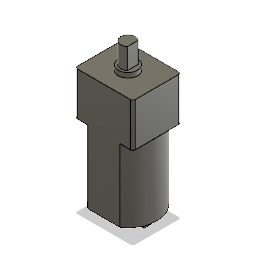
Motorized bigjoint (Autodesk Fusion 360 archive; units mm, degrees)
design "VE508 Small Gear Motor"
Autodesk Fusion 360 part; units mm, degrees
note: some values were not read from the file. Set by a fixed rule: which sketch regions a step uses.
(part 1 of 2)
sketch "Sketch1" plane through (0, 0, 0) normal (0, 1, 0) x (1, 0, 0) in component "Motor"
  line L0 (6, 5) -> (-6, 5)
  line L1 (-6, 5) -> (-6, -5)
  line L2 (-6, -5) -> (6, -5)
  line L3 (6, -5) -> (6, 5)
  line L4 (6, 5) -> (-6, -5) construction
  line L5 (-6, 5) -> (6, -5) construction
  dimension "d1" = 10
  dimension "d2" = 12
  constraint perpendicular L0 L1
  constraint parallel L0 L2
  constraint parallel L1 L3
  constraint horizontal L0
  constraint coincident L4 origin
  constraint coincident L5 origin
  measures "d1" distance of L0.end L1.end
  measures "d2" distance of L0.start L0.end
extrude "Extrude1" add sketch "Sketch1" against normal blind 9 makes body 1 in component "Motor"
sketch "Sketch2" plane through (0, -9, 0) normal (0, -1, 0) x (1, 0, 0) in component "Motor"
  line L0 (6, -5) -> (6, 5)
  line L1 (6, 5) -> (-6, 5)
  line L2 (-6, 5) -> (-6, -5)
  line L3 (-6, -5) -> (6, -5)
  circle A0 centre (0, 0) radius 6
  constraint coincident A0.centre origin
  constraint tangent L0 A0
extrude "Extrude2" add sketch "Sketch2" along normal blind 15 contours L1 L3 A0 bodies 1 in component "Motor"
sketch "Sketch3" plane through (0, -24, 0) normal (0, -1, 0) x (1, 0, 0) in component "Motor"
  arc A0 (3.3166, -5) -> (3.3166, 5) centre (0, 0) ccw
  line L0 (3.3166, 5) -> (-3.3166, 5)
  arc A1 (-3.3166, 5) -> (-3.3166, -5) centre (0, 0) ccw
  line L1 (-3.3166, -5) -> (3.3166, -5)
  circle A2 centre (0, 0) radius 2.5
  line L2 (-4, 0) -> (4, 0) construction
  line L3 (0, 5) -> (0, -5) construction
  line L4 (-4, 0.75) -> (-3.65, 0.75)
  line L5 (-3.65, 0.75) -> (-3.65, -0.75)
  line L6 (-3.65, -0.75) -> (-4, -0.75)
  line L7 (-4, -0.75) -> (-4, 0.75)
  line L8 (3.65, -0.75) -> (4, -0.75)
  line L9 (4, -0.75) -> (4, 0.75)
  line L10 (3.65, 0.75) -> (3.65, -0.75)
  line L11 (4, 0.75) -> (3.65, 0.75)
  dimension "d7" = 5
  dimension "d10" = 8
  dimension "d11" = 0.35
  dimension "d12" = 1.5
  constraint concentric A0 A2
  constraint horizontal L2
  constraint coincident A0.centre L2
  constraint midpoint L0 L3.start
  constraint midpoint L1 L3.end
  constraint symmetric L2.start L2.end L3
  constraint horizontal L4
  constraint vertical L5
  constraint horizontal L6
  constraint vertical L7
  constraint coincident L2.start L7
  constraint symmetric L2 L4 L6
  constraint symmetric L3 L4.start L9.end
  constraint symmetric L3 L4.end L10.start
  constraint symmetric L3 L5.end L8.start
  constraint symmetric L3 L6.end L8.end
  measures "d7" diameter of A2
  measures "d10" distance of L2.start L2.end
  measures "d11" distance of L5.end L6.end
  measures "d12" distance of L4.start L6.end
extrude "Extrude4" add sketch "Sketch3" along normal blind 2 contours L4 L5 L6 L7 | L8 L9 L10 L11 bodies 1 in component "Motor"
extrude "Extrude3" add sketch "Sketch3" along normal blind 1 contours A2 bodies 1 in component "Motor"
fillet "Fillet1" radius 0.5 4 edges at (6, -4.5, -5) (-6, -4.5, -5) (-6, -4.5, 5) (6, -4.5, 5) on bodies 1 in component "Motor"
sketch "Sketch4" plane through (0, 0, 0) normal (0, 1, 0) x (-1, 0, 0) in component "Motor"
  arc A0 (-5.5, 5) -> (-6, 4.5) centre (-5.5, 4.5) ccw
  line L0 (-6, 4.5) -> (-6, -4.5)
  arc A1 (-6, -4.5) -> (-5.5, -5) centre (-5.5, -4.5) ccw
  line L1 (-5.5, -5) -> (5.5, -5)
  arc A2 (5.5, -5) -> (6, -4.5) centre (5.5, -4.5) ccw
  line L2 (6, -4.5) -> (6, 4.5)
  arc A3 (6, 4.5) -> (5.5, 5) centre (5.5, 4.5) ccw
  line L3 (5.5, 5) -> (-5.5, 5)
  circle A4 centre (0, 0) radius 2
  dimension "d16" = 4
  constraint coincident A4.centre origin
  measures "d16" diameter of A4
extrude "Extrude5" add sketch "Sketch4" along normal blind 1 contours A4 bodies 1 in component "Motor"
sketch "Sketch5" plane through (0, 1, 0) normal (0, 1, 0) x (-1, 0, 0) in component "Motor"
  circle A0 centre (0, 0) radius 2
  circle A1 centre (0, 0) radius 1.5
  line L0 (-1, -1.118) -> (-1, 1.118)
  line L1 (3.3166, -5) -> (-3.3166, -5) construction
  line L2 (5.5, 5) -> (-5.5, 5) construction
  line L3 (1.5, -5) -> (1.5, 5) construction
  dimension "d19" = 3
  dimension "d20" = 2.5
  constraint concentric A0 A1
  constraint coincident A1 L0.start
  constraint coincident A1 L0.end
  constraint coincident L1 L3.start
  constraint coincident L2 L3.end
  constraint tangent A1 L3
  constraint perpendicular L2 L3
  measures "d19" diameter of A1
  measures "d20" distance of L0 L3
extrude "Extrude6" add sketch "Sketch5" along normal blind 4.3 separate body contours A1 L0 picked at (-0.4625, 0.4564) makes body 2 in component "Motor"
copy_body "CutPasteBodies1" bodies 2 removing the originals makes body 3 in component "Rotor"
component "Motor" placed x (1, 0, 0) y (0, 1, 0) z (0, 0, 1) at (0, 0, 0)
component "Rotor" placed x (1, 0, 0) y (0, 1, 0) z (0, 0, 1) at (0, 0, 0)

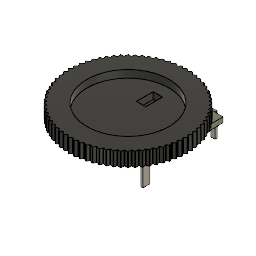
design "B503 Dial Potentiometer"
Autodesk Fusion 360 part; units mm, degrees
sketch "Sketch1" plane through (0, 0, 0) normal (0, 0, 1) x (1, 0, 0) in component "Knob"
  circle A0 centre (0, 0) radius 8
  circle A1 centre (0, 0) radius 7.75
  line L0 (0, 0) -> (8, 0) construction
  line L1 (7.7444, 0.2955) -> (7.9999, 0.04)
  line L2 (7.7444, -0.2955) -> (7.9999, -0.04)
  line L3 (7.7407, 0.3806) -> (7.9729, 0.6574)
  line L4 (7.6891, 0.9694) -> (7.966, 0.7371)
  line L5 (7.678, 1.0537) -> (7.8853, 1.3498)
  line L6 (7.5754, 1.6358) -> (7.8714, 1.4286)
  line L7 (7.557, 1.7189) -> (7.7377, 2.0319)
  line L8 (7.404, 2.2899) -> (7.717, 2.1092)
  line L9 (7.3784, 2.371) -> (7.5311, 2.6985)
  line L10 (7.1762, 2.9264) -> (7.5038, 2.7737)
  line L11 (7.1437, 3.0051) -> (7.2673, 3.3447)
  line L12 (6.8939, 3.5408) -> (7.2335, 3.4172)
  line L13 (6.8546, 3.6162) -> (6.9481, 3.9653)
  line L14 (6.559, 4.1281) -> (6.9081, 4.0346)
  line L15 (6.5133, 4.1999) -> (6.5761, 4.5558)
  line L16 (6.1743, 4.6841) -> (6.5302, 4.6213)
  line L17 (6.1225, 4.7516) -> (6.154, 5.1116)
  line L18 (5.7426, 5.2044) -> (6.1026, 5.1729)
  line L19 (5.6851, 5.2671) -> (5.6851, 5.6285)
  line L20 (5.2671, 5.6851) -> (5.6285, 5.6851)
  line L21 (5.2044, 5.7426) -> (5.1729, 6.1026)
  line L22 (4.7516, 6.1225) -> (5.1116, 6.154)
  line L23 (4.6841, 6.1743) -> (4.6213, 6.5302)
  line L24 (4.1999, 6.5133) -> (4.5558, 6.5761)
  line L25 (4.1281, 6.559) -> (4.0346, 6.9081)
  line L26 (3.6162, 6.8546) -> (3.9653, 6.9481)
  line L27 (3.5408, 6.8939) -> (3.4172, 7.2335)
  line L28 (3.0051, 7.1437) -> (3.3447, 7.2673)
  line L29 (2.9264, 7.1762) -> (2.7737, 7.5038)
  line L30 (2.371, 7.3784) -> (2.6985, 7.5311)
  line L31 (2.2899, 7.404) -> (2.1092, 7.717)
  line L32 (1.7189, 7.557) -> (2.0319, 7.7377)
  line L33 (1.6358, 7.5754) -> (1.4286, 7.8714)
  line L34 (1.0537, 7.678) -> (1.3498, 7.8853)
  line L35 (0.9694, 7.6891) -> (0.7371, 7.966)
  line L36 (0.3806, 7.7407) -> (0.6574, 7.9729)
  line L37 (0.2955, 7.7444) -> (0.04, 7.9999)
  line L38 (-0.2955, 7.7444) -> (-0.04, 7.9999)
  line L39 (-0.3806, 7.7407) -> (-0.6574, 7.9729)
  line L40 (-0.9694, 7.6891) -> (-0.7371, 7.966)
  line L41 (-1.0537, 7.678) -> (-1.3498, 7.8853)
  line L42 (-1.6358, 7.5754) -> (-1.4286, 7.8714)
  line L43 (-1.7189, 7.557) -> (-2.0319, 7.7377)
  line L44 (-2.2899, 7.404) -> (-2.1092, 7.717)
  line L45 (-2.371, 7.3784) -> (-2.6985, 7.5311)
  line L46 (-2.9264, 7.1762) -> (-2.7737, 7.5038)
  line L47 (-3.0051, 7.1437) -> (-3.3447, 7.2673)
  line L48 (-3.5408, 6.8939) -> (-3.4172, 7.2335)
  line L49 (-3.6162, 6.8546) -> (-3.9653, 6.9481)
  line L50 (-4.1281, 6.559) -> (-4.0346, 6.9081)
  line L51 (-4.1999, 6.5133) -> (-4.5558, 6.5761)
  line L52 (-4.6841, 6.1743) -> (-4.6213, 6.5302)
  line L53 (-4.7516, 6.1225) -> (-5.1116, 6.154)
  line L54 (-5.2044, 5.7426) -> (-5.1729, 6.1026)
  line L55 (-5.2671, 5.6851) -> (-5.6285, 5.6851)
  line L56 (-5.6851, 5.2671) -> (-5.6851, 5.6285)
  line L57 (-5.7426, 5.2044) -> (-6.1026, 5.1729)
  line L58 (-6.1225, 4.7516) -> (-6.154, 5.1116)
  line L59 (-6.1743, 4.6841) -> (-6.5302, 4.6213)
  line L60 (-6.5133, 4.1999) -> (-6.5761, 4.5558)
  line L61 (-6.559, 4.1281) -> (-6.9081, 4.0346)
  line L62 (-6.8546, 3.6162) -> (-6.9481, 3.9653)
  line L63 (-6.8939, 3.5408) -> (-7.2335, 3.4172)
  line L64 (-7.1437, 3.0051) -> (-7.2673, 3.3447)
  line L65 (-7.1762, 2.9264) -> (-7.5038, 2.7737)
  line L66 (-7.3784, 2.371) -> (-7.5311, 2.6985)
  line L67 (-7.404, 2.2899) -> (-7.717, 2.1092)
  line L68 (-7.557, 1.7189) -> (-7.7377, 2.0319)
  line L69 (-7.5754, 1.6358) -> (-7.8714, 1.4286)
  line L70 (-7.678, 1.0537) -> (-7.8853, 1.3498)
  line L71 (-7.6891, 0.9694) -> (-7.966, 0.7371)
  line L72 (-7.7407, 0.3806) -> (-7.9729, 0.6574)
  line L73 (-7.7444, 0.2955) -> (-7.9999, 0.04)
  line L74 (-7.7444, -0.2955) -> (-7.9999, -0.04)
  line L75 (-7.7407, -0.3806) -> (-7.9729, -0.6574)
  line L76 (-7.6891, -0.9694) -> (-7.966, -0.7371)
  line L77 (-7.678, -1.0537) -> (-7.8853, -1.3498)
  line L78 (-7.5754, -1.6358) -> (-7.8714, -1.4286)
  line L79 (-7.557, -1.7189) -> (-7.7377, -2.0319)
  line L80 (-7.404, -2.2899) -> (-7.717, -2.1092)
  line L81 (-7.3784, -2.371) -> (-7.5311, -2.6985)
  line L82 (-7.1762, -2.9264) -> (-7.5038, -2.7737)
  line L83 (-7.1437, -3.0051) -> (-7.2673, -3.3447)
  line L84 (-6.8939, -3.5408) -> (-7.2335, -3.4172)
  line L85 (-6.8546, -3.6162) -> (-6.9481, -3.9653)
  line L86 (-6.559, -4.1281) -> (-6.9081, -4.0346)
  line L87 (-6.5133, -4.1999) -> (-6.5761, -4.5558)
  line L88 (-6.1743, -4.6841) -> (-6.5302, -4.6213)
  line L89 (-6.1225, -4.7516) -> (-6.154, -5.1116)
  line L90 (-5.7426, -5.2044) -> (-6.1026, -5.1729)
  line L91 (-5.6851, -5.2671) -> (-5.6851, -5.6285)
  line L92 (-5.2671, -5.6851) -> (-5.6285, -5.6851)
  line L93 (-5.2044, -5.7426) -> (-5.1729, -6.1026)
  line L94 (-4.7516, -6.1225) -> (-5.1116, -6.154)
  line L95 (-4.6841, -6.1743) -> (-4.6213, -6.5302)
  line L96 (-4.1999, -6.5133) -> (-4.5558, -6.5761)
  line L97 (-4.1281, -6.559) -> (-4.0346, -6.9081)
  line L98 (-3.6162, -6.8546) -> (-3.9653, -6.9481)
  line L99 (-3.5408, -6.8939) -> (-3.4172, -7.2335)
  line L100 (-3.0051, -7.1437) -> (-3.3447, -7.2673)
  line L101 (-2.9264, -7.1762) -> (-2.7737, -7.5038)
  line L102 (-2.371, -7.3784) -> (-2.6985, -7.5311)
  line L103 (-2.2899, -7.404) -> (-2.1092, -7.717)
  line L104 (-1.7189, -7.557) -> (-2.0319, -7.7377)
  line L105 (-1.6358, -7.5754) -> (-1.4286, -7.8714)
  line L106 (-1.0537, -7.678) -> (-1.3498, -7.8853)
  line L107 (-0.9694, -7.6891) -> (-0.7371, -7.966)
  line L108 (-0.3806, -7.7407) -> (-0.6574, -7.9729)
  line L109 (-0.2955, -7.7444) -> (-0.04, -7.9999)
  line L110 (0.2955, -7.7444) -> (0.04, -7.9999)
  line L111 (0.3806, -7.7407) -> (0.6574, -7.9729)
  line L112 (0.9694, -7.6891) -> (0.7371, -7.966)
  line L113 (1.0537, -7.678) -> (1.3498, -7.8853)
  line L114 (1.6358, -7.5754) -> (1.4286, -7.8714)
  line L115 (1.7189, -7.557) -> (2.0319, -7.7377)
  line L116 (2.2899, -7.404) -> (2.1092, -7.717)
  line L117 (2.371, -7.3784) -> (2.6985, -7.5311)
  line L118 (2.9264, -7.1762) -> (2.7737, -7.5038)
  line L119 (3.0051, -7.1437) -> (3.3447, -7.2673)
  line L120 (3.5408, -6.8939) -> (3.4172, -7.2335)
  line L121 (3.6162, -6.8546) -> (3.9653, -6.9481)
  line L122 (4.1281, -6.559) -> (4.0346, -6.9081)
  line L123 (4.1999, -6.5133) -> (4.5558, -6.5761)
  line L124 (4.6841, -6.1743) -> (4.6213, -6.5302)
  line L125 (4.7516, -6.1225) -> (5.1116, -6.154)
  line L126 (5.2044, -5.7426) -> (5.1729, -6.1026)
  line L127 (5.2671, -5.6851) -> (5.6285, -5.6851)
  line L128 (5.6851, -5.2671) -> (5.6851, -5.6285)
  line L129 (5.7426, -5.2044) -> (6.1026, -5.1729)
  line L130 (6.1225, -4.7516) -> (6.154, -5.1116)
  line L131 (6.1743, -4.6841) -> (6.5302, -4.6213)
  line L132 (6.5133, -4.1999) -> (6.5761, -4.5558)
  line L133 (6.559, -4.1281) -> (6.9081, -4.0346)
  line L134 (6.8546, -3.6162) -> (6.9481, -3.9653)
  line L135 (6.8939, -3.5408) -> (7.2335, -3.4172)
  line L136 (7.1437, -3.0051) -> (7.2673, -3.3447)
  line L137 (7.1762, -2.9264) -> (7.5038, -2.7737)
  line L138 (7.3784, -2.371) -> (7.5311, -2.6985)
  line L139 (7.404, -2.2899) -> (7.717, -2.1092)
  line L140 (7.557, -1.7189) -> (7.7377, -2.0319)
  line L141 (7.5754, -1.6358) -> (7.8714, -1.4286)
  line L142 (7.678, -1.0537) -> (7.8853, -1.3498)
  line L143 (7.6891, -0.9694) -> (7.966, -0.7371)
  line L144 (7.7407, -0.3806) -> (7.9729, -0.6574)
  dimension "d1" = 16
  dimension "d4" = 15.5
  dimension "d5" = 90
  dimension "d7" = 360
  dimension "d8" = 0.08
  dimension "d62" = 0
  dimension "d63" = 0
  dimension "d64" = 0
  dimension "d65" = 0
  constraint coincident A0.centre A1.centre
  constraint horizontal L0
  constraint coincident A1 L1.start
  constraint coincident A1 L2.start
  constraint symmetric L0 L1 L2
  constraint coincident A0 L2.end
  constraint coincident A0 L1.end
  constraint coincident A0 L0.end
  measures "d1" diameter of A0
  measures "d4" diameter of A1
  measures "d5" angle of L1 L2
  measures "d8" distance of L2.end L1.end
extrude "Extrude2" add sketch "Sketch1" along normal blind 1.9 contours A0 A1 L1 L2 | A0 A1 L3 L4 | A1 | A0 A1 L143 L144 | A0 A1 L5 L6 | A0 A1 L141 L142 | A0 A1 L7 L8 | A0 A1 L139 L140 | A0 A1 L9 L10 | A0 A1 L137 L138 | A0 A1 L11 L12 | A0 A1 L135 L136 | A0 A1 L13 L14 | A0 A1 L133 L134 | A0 A1 L15 L16 | A0 A1 L131 L132 | A0 A1 L17 L18 | A0 A1 L129 L130 | A0 A1 L19 L20 | A0 A1 L127 L128 | A0 A1 L21 L22 | A0 A1 L125 L126 | A0 A1 L23 L24 | A0 A1 L123 L124 | A0 A1 L25 L26 | A0 A1 L121 L122 | A0 A1 L27 L28 | A0 A1 L119 L120 | A0 A1 L29 L30 | A0 A1 L117 L118 | A0 A1 L31 L32 | A0 A1 L115 L116 | A0 A1 L33 L34 | A0 A1 L113 L114 | A0 A1 L35 L36 | A0 A1 L111 L112 | A0 A1 L37 L38 | A0 A1 L109 L110 | A0 A1 L39 L40 | A0 A1 L107 L108 | A0 A1 L41 L42 | A0 A1 L105 L106 | A0 A1 L43 L44 | A0 A1 L103 L104 | A0 A1 L45 L46 | A0 A1 L101 L102 | A0 A1 L47 L48 | A0 A1 L99 L100 | A0 A1 L49 L50 | A0 A1 L97 L98 | A0 A1 L51 L52 | A0 A1 L95 L96 | A0 A1 L53 L54 | A0 A1 L93 L94 | A0 A1 L55 L56 | A0 A1 L91 L92 | A0 A1 L57 L58 | A0 A1 L89 L90 | A0 A1 L59 L60 | A0 A1 L87 L88 | A0 A1 L61 L62 | A0 A1 L85 L86 | A0 A1 L63 L64 | A0 A1 L83 L84 | A0 A1 L65 L66 | A0 A1 L81 L82 | A0 A1 L67 L68 | A0 A1 L79 L80 | A0 A1 L69 L70 | A0 A1 L77 L78 | A0 A1 L71 L72 | A0 A1 L75 L76 | A0 A1 L73 L74 makes body 1 in component "Knob"
sketch "Sketch1 (1)" plane through (0, 0, 1.9) normal (0, 0, 1) x (-1, 0, 0) in component "Knob"
  line L0 (-7.7444, 0.2955) -> (-7.9999, 0.04)
  arc A0 (-7.9999, 0.04) -> (-7.9999, -0.04) centre (0, 0) ccw
  line L1 (-7.9999, -0.04) -> (-7.7444, -0.2955)
  arc A1 (-7.7444, -0.2955) -> (-7.7407, -0.3806) centre (0, 0) ccw
  line L2 (-7.7407, -0.3806) -> (-7.9729, -0.6574)
  arc A2 (-7.9729, -0.6574) -> (-7.966, -0.7371) centre (0, 0) ccw
  line L3 (-7.966, -0.7371) -> (-7.6891, -0.9694)
  arc A3 (-7.6891, -0.9694) -> (-7.678, -1.0537) centre (0, 0) ccw
  line L4 (-7.678, -1.0537) -> (-7.8853, -1.3498)
  arc A4 (-7.8853, -1.3498) -> (-7.8714, -1.4286) centre (0, 0) ccw
  line L5 (-7.8714, -1.4286) -> (-7.5754, -1.6358)
  arc A5 (-7.5754, -1.6358) -> (-7.557, -1.7189) centre (0, 0) ccw
  line L6 (-7.557, -1.7189) -> (-7.7377, -2.0319)
  arc A6 (-7.7377, -2.0319) -> (-7.717, -2.1092) centre (0, 0) ccw
  line L7 (-7.717, -2.1092) -> (-7.404, -2.2899)
  arc A7 (-7.404, -2.2899) -> (-7.3784, -2.371) centre (0, 0) ccw
  line L8 (-7.3784, -2.371) -> (-7.5311, -2.6985)
  arc A8 (-7.5311, -2.6985) -> (-7.5038, -2.7737) centre (0, 0) ccw
  line L9 (-7.5038, -2.7737) -> (-7.1762, -2.9264)
  arc A9 (-7.1762, -2.9264) -> (-7.1437, -3.0051) centre (0, 0) ccw
  line L10 (-7.1437, -3.0051) -> (-7.2673, -3.3447)
  arc A10 (-7.2673, -3.3447) -> (-7.2335, -3.4172) centre (0, 0) ccw
  line L11 (-7.2335, -3.4172) -> (-6.8939, -3.5408)
  arc A11 (-6.8939, -3.5408) -> (-6.8546, -3.6162) centre (0, 0) ccw
  line L12 (-6.8546, -3.6162) -> (-6.9481, -3.9653)
  arc A12 (-6.9481, -3.9653) -> (-6.9081, -4.0346) centre (0, 0) ccw
  line L13 (-6.9081, -4.0346) -> (-6.559, -4.1281)
  arc A13 (-6.559, -4.1281) -> (-6.5133, -4.1999) centre (0, 0) ccw
  line L14 (-6.5133, -4.1999) -> (-6.5761, -4.5558)
  arc A14 (-6.5761, -4.5558) -> (-6.5302, -4.6213) centre (0, 0) ccw
  line L15 (-6.5302, -4.6213) -> (-6.1743, -4.6841)
  arc A15 (-6.1743, -4.6841) -> (-6.1225, -4.7516) centre (0, 0) ccw
  line L16 (-6.1225, -4.7516) -> (-6.154, -5.1116)
  arc A16 (-6.154, -5.1116) -> (-6.1026, -5.1729) centre (0, 0) ccw
  line L17 (-6.1026, -5.1729) -> (-5.7426, -5.2044)
  arc A17 (-5.7426, -5.2044) -> (-5.6851, -5.2671) centre (0, 0) ccw
  line L18 (-5.6851, -5.2671) -> (-5.6851, -5.6285)
  arc A18 (-5.6851, -5.6285) -> (-5.6285, -5.6851) centre (0, 0) ccw
  line L19 (-5.6285, -5.6851) -> (-5.2671, -5.6851)
  arc A19 (-5.2671, -5.6851) -> (-5.2044, -5.7426) centre (0, 0) ccw
  line L20 (-5.2044, -5.7426) -> (-5.1729, -6.1026)
  arc A20 (-5.1729, -6.1026) -> (-5.1116, -6.154) centre (0, 0) ccw
  line L21 (-5.1116, -6.154) -> (-4.7516, -6.1225)
  arc A21 (-4.7516, -6.1225) -> (-4.6841, -6.1743) centre (0, 0) ccw
  line L22 (-4.6841, -6.1743) -> (-4.6213, -6.5302)
  arc A22 (-4.6213, -6.5302) -> (-4.5558, -6.5761) centre (0, 0) ccw
  line L23 (-4.5558, -6.5761) -> (-4.1999, -6.5133)
  arc A23 (-4.1999, -6.5133) -> (-4.1281, -6.559) centre (0, 0) ccw
  line L24 (-4.1281, -6.559) -> (-4.0346, -6.9081)
  arc A24 (-4.0346, -6.9081) -> (-3.9653, -6.9481) centre (0, 0) ccw
  line L25 (-3.9653, -6.9481) -> (-3.6162, -6.8546)
  arc A25 (-3.6162, -6.8546) -> (-3.5408, -6.8939) centre (0, 0) ccw
  line L26 (-3.5408, -6.8939) -> (-3.4172, -7.2335)
  arc A26 (-3.4172, -7.2335) -> (-3.3447, -7.2673) centre (0, 0) ccw
  line L27 (-3.3447, -7.2673) -> (-3.0051, -7.1437)
  arc A27 (-3.0051, -7.1437) -> (-2.9264, -7.1762) centre (0, 0) ccw
  line L28 (-2.9264, -7.1762) -> (-2.7737, -7.5038)
  arc A28 (-2.7737, -7.5038) -> (-2.6985, -7.5311) centre (0, 0) ccw
  line L29 (-2.6985, -7.5311) -> (-2.371, -7.3784)
  arc A29 (-2.371, -7.3784) -> (-2.2899, -7.404) centre (0, 0) ccw
  line L30 (-2.2899, -7.404) -> (-2.1092, -7.717)
  arc A30 (-2.1092, -7.717) -> (-2.0319, -7.7377) centre (0, 0) ccw
  line L31 (-2.0319, -7.7377) -> (-1.7189, -7.557)
  arc A31 (-1.7189, -7.557) -> (-1.6358, -7.5754) centre (0, 0) ccw
  line L32 (-1.6358, -7.5754) -> (-1.4286, -7.8714)
  arc A32 (-1.4286, -7.8714) -> (-1.3498, -7.8853) centre (0, 0) ccw
  line L33 (-1.3498, -7.8853) -> (-1.0537, -7.678)
  arc A33 (-1.0537, -7.678) -> (-0.9694, -7.6891) centre (0, 0) ccw
  line L34 (-0.9694, -7.6891) -> (-0.7371, -7.966)
  arc A34 (-0.7371, -7.966) -> (-0.6574, -7.9729) centre (0, 0) ccw
  line L35 (-0.6574, -7.9729) -> (-0.3806, -7.7407)
  arc A35 (-0.3806, -7.7407) -> (-0.2955, -7.7444) centre (0, 0) ccw
  line L36 (-0.2955, -7.7444) -> (-0.04, -7.9999)
  arc A36 (-0.04, -7.9999) -> (0.04, -7.9999) centre (0, 0) ccw
  line L37 (0.04, -7.9999) -> (0.2955, -7.7444)
  arc A37 (0.2955, -7.7444) -> (0.3806, -7.7407) centre (0, 0) ccw
  line L38 (0.3806, -7.7407) -> (0.6574, -7.9729)
  arc A38 (0.6574, -7.9729) -> (0.7371, -7.966) centre (0, 0) ccw
  line L39 (0.7371, -7.966) -> (0.9694, -7.6891)
  arc A39 (0.9694, -7.6891) -> (1.0537, -7.678) centre (0, 0) ccw
  line L40 (1.0537, -7.678) -> (1.3498, -7.8853)
  arc A40 (1.3498, -7.8853) -> (1.4286, -7.8714) centre (0, 0) ccw
  line L41 (1.4286, -7.8714) -> (1.6358, -7.5754)
  arc A41 (1.6358, -7.5754) -> (1.7189, -7.557) centre (0, 0) ccw
  line L42 (1.7189, -7.557) -> (2.0319, -7.7377)
  arc A42 (2.0319, -7.7377) -> (2.1092, -7.717) centre (0, 0) ccw
  line L43 (2.1092, -7.717) -> (2.2899, -7.404)
  arc A43 (2.2899, -7.404) -> (2.371, -7.3784) centre (0, 0) ccw
  line L44 (2.371, -7.3784) -> (2.6985, -7.5311)
  arc A44 (2.6985, -7.5311) -> (2.7737, -7.5038) centre (0, 0) ccw
  line L45 (2.7737, -7.5038) -> (2.9264, -7.1762)
  arc A45 (2.9264, -7.1762) -> (3.0051, -7.1437) centre (0, 0) ccw
  line L46 (3.0051, -7.1437) -> (3.3447, -7.2673)
  arc A46 (3.3447, -7.2673) -> (3.4172, -7.2335) centre (0, 0) ccw
  line L47 (3.4172, -7.2335) -> (3.5408, -6.8939)
  arc A47 (3.5408, -6.8939) -> (3.6162, -6.8546) centre (0, 0) ccw
  line L48 (3.6162, -6.8546) -> (3.9653, -6.9481)
  arc A48 (3.9653, -6.9481) -> (4.0346, -6.9081) centre (0, 0) ccw
  line L49 (4.0346, -6.9081) -> (4.1281, -6.559)
  arc A49 (4.1281, -6.559) -> (4.1999, -6.5133) centre (0, 0) ccw
  line L50 (4.1999, -6.5133) -> (4.5558, -6.5761)
  arc A50 (4.5558, -6.5761) -> (4.6213, -6.5302) centre (0, 0) ccw
  line L51 (4.6213, -6.5302) -> (4.6841, -6.1743)
  arc A51 (4.6841, -6.1743) -> (4.7516, -6.1225) centre (0, 0) ccw
  line L52 (4.7516, -6.1225) -> (5.1116, -6.154)
  arc A52 (5.1116, -6.154) -> (5.1729, -6.1026) centre (0, 0) ccw
  line L53 (5.1729, -6.1026) -> (5.2044, -5.7426)
  arc A53 (5.2044, -5.7426) -> (5.2671, -5.6851) centre (0, 0) ccw
  line L54 (5.2671, -5.6851) -> (5.6285, -5.6851)
  arc A54 (5.6285, -5.6851) -> (5.6851, -5.6285) centre (0, 0) ccw
  line L55 (5.6851, -5.6285) -> (5.6851, -5.2671)
  arc A55 (5.6851, -5.2671) -> (5.7426, -5.2044) centre (0, 0) ccw
  line L56 (5.7426, -5.2044) -> (6.1026, -5.1729)
  arc A56 (6.1026, -5.1729) -> (6.154, -5.1116) centre (0, 0) ccw
  line L57 (6.154, -5.1116) -> (6.1225, -4.7516)
  arc A57 (6.1225, -4.7516) -> (6.1743, -4.6841) centre (0, 0) ccw
  line L58 (6.1743, -4.6841) -> (6.5302, -4.6213)
  arc A58 (6.5302, -4.6213) -> (6.5761, -4.5558) centre (0, 0) ccw
  line L59 (6.5761, -4.5558) -> (6.5133, -4.1999)
  arc A59 (6.5133, -4.1999) -> (6.559, -4.1281) centre (0, 0) ccw
  line L60 (6.559, -4.1281) -> (6.9081, -4.0346)
  arc A60 (6.9081, -4.0346) -> (6.9481, -3.9653) centre (0, 0) ccw
  line L61 (6.9481, -3.9653) -> (6.8546, -3.6162)
  arc A61 (6.8546, -3.6162) -> (6.8939, -3.5408) centre (0, 0) ccw
  line L62 (6.8939, -3.5408) -> (7.2335, -3.4172)
  arc A62 (7.2335, -3.4172) -> (7.2673, -3.3447) centre (0, 0) ccw
  line L63 (7.2673, -3.3447) -> (7.1437, -3.0051)
  arc A63 (7.1437, -3.0051) -> (7.1762, -2.9264) centre (0, 0) ccw
  line L64 (7.1762, -2.9264) -> (7.5038, -2.7737)
  arc A64 (7.5038, -2.7737) -> (7.5311, -2.6985) centre (0, 0) ccw
  line L65 (7.5311, -2.6985) -> (7.3784, -2.371)
  arc A65 (7.3784, -2.371) -> (7.404, -2.2899) centre (0, 0) ccw
  line L66 (7.404, -2.2899) -> (7.717, -2.1092)
  arc A66 (7.717, -2.1092) -> (7.7377, -2.0319) centre (0, 0) ccw
  line L67 (7.7377, -2.0319) -> (7.557, -1.7189)
  arc A67 (7.557, -1.7189) -> (7.5754, -1.6358) centre (0, 0) ccw
  line L68 (7.5754, -1.6358) -> (7.8714, -1.4286)
  arc A68 (7.8714, -1.4286) -> (7.8853, -1.3498) centre (0, 0) ccw
  line L69 (7.8853, -1.3498) -> (7.678, -1.0537)
  arc A69 (7.678, -1.0537) -> (7.6891, -0.9694) centre (0, 0) ccw
  line L70 (7.6891, -0.9694) -> (7.966, -0.7371)
  arc A70 (7.966, -0.7371) -> (7.9729, -0.6574) centre (0, 0) ccw
  line L71 (7.9729, -0.6574) -> (7.7407, -0.3806)
  arc A71 (7.7407, -0.3806) -> (7.7444, -0.2955) centre (0, 0) ccw
  line L72 (7.7444, -0.2955) -> (7.9999, -0.04)
  arc A72 (7.9999, -0.04) -> (7.9999, 0.04) centre (0, 0) ccw
  line L73 (7.9999, 0.04) -> (7.7444, 0.2955)
  arc A73 (7.7444, 0.2955) -> (7.7407, 0.3806) centre (0, 0) ccw
  line L74 (7.7407, 0.3806) -> (7.9729, 0.6574)
  arc A74 (7.9729, 0.6574) -> (7.966, 0.7371) centre (0, 0) ccw
  line L75 (7.966, 0.7371) -> (7.6891, 0.9694)
  arc A75 (7.6891, 0.9694) -> (7.678, 1.0537) centre (0, 0) ccw
  line L76 (7.678, 1.0537) -> (7.8853, 1.3498)
  arc A76 (7.8853, 1.3498) -> (7.8714, 1.4286) centre (0, 0) ccw
  line L77 (7.8714, 1.4286) -> (7.5754, 1.6358)
  arc A77 (7.5754, 1.6358) -> (7.557, 1.7189) centre (0, 0) ccw
  line L78 (7.557, 1.7189) -> (7.7377, 2.0319)
  arc A78 (7.7377, 2.0319) -> (7.717, 2.1092) centre (0, 0) ccw
  line L79 (7.717, 2.1092) -> (7.404, 2.2899)
  arc A79 (7.404, 2.2899) -> (7.3784, 2.371) centre (0, 0) ccw
  line L80 (7.3784, 2.371) -> (7.5311, 2.6985)
  arc A80 (7.5311, 2.6985) -> (7.5038, 2.7737) centre (0, 0) ccw
  line L81 (7.5038, 2.7737) -> (7.1762, 2.9264)
  arc A81 (7.1762, 2.9264) -> (7.1437, 3.0051) centre (0, 0) ccw
  line L82 (7.1437, 3.0051) -> (7.2673, 3.3447)
  arc A82 (7.2673, 3.3447) -> (7.2335, 3.4172) centre (0, 0) ccw
  line L83 (7.2335, 3.4172) -> (6.8939, 3.5408)
  arc A83 (6.8939, 3.5408) -> (6.8546, 3.6162) centre (0, 0) ccw
  line L84 (6.8546, 3.6162) -> (6.9481, 3.9653)
  arc A84 (6.9481, 3.9653) -> (6.9081, 4.0346) centre (0, 0) ccw
  line L85 (6.9081, 4.0346) -> (6.559, 4.1281)
  arc A85 (6.559, 4.1281) -> (6.5133, 4.1999) centre (0, 0) ccw
  line L86 (6.5133, 4.1999) -> (6.5761, 4.5558)
  arc A86 (6.5761, 4.5558) -> (6.5302, 4.6213) centre (0, 0) ccw
  line L87 (6.5302, 4.6213) -> (6.1743, 4.6841)
  arc A87 (6.1743, 4.6841) -> (6.1225, 4.7516) centre (0, 0) ccw
  line L88 (6.1225, 4.7516) -> (6.154, 5.1116)
  arc A88 (6.154, 5.1116) -> (6.1026, 5.1729) centre (0, 0) ccw
  line L89 (6.1026, 5.1729) -> (5.7426, 5.2044)
  arc A89 (5.7426, 5.2044) -> (5.6851, 5.2671) centre (0, 0) ccw
  line L90 (5.6851, 5.2671) -> (5.6851, 5.6285)
  arc A90 (5.6851, 5.6285) -> (5.6285, 5.6851) centre (0, 0) ccw
  line L91 (5.6285, 5.6851) -> (5.2671, 5.6851)
  arc A91 (5.2671, 5.6851) -> (5.2044, 5.7426) centre (0, 0) ccw
  line L92 (5.2044, 5.7426) -> (5.1729, 6.1026)
  arc A92 (5.1729, 6.1026) -> (5.1116, 6.154) centre (0, 0) ccw
  line L93 (5.1116, 6.154) -> (4.7516, 6.1225)
  arc A93 (4.7516, 6.1225) -> (4.6841, 6.1743) centre (0, 0) ccw
  line L94 (4.6841, 6.1743) -> (4.6213, 6.5302)
  arc A94 (4.6213, 6.5302) -> (4.5558, 6.5761) centre (0, 0) ccw
  line L95 (4.5558, 6.5761) -> (4.1999, 6.5133)
  arc A95 (4.1999, 6.5133) -> (4.1281, 6.559) centre (0, 0) ccw
  line L96 (4.1281, 6.559) -> (4.0346, 6.9081)
  arc A96 (4.0346, 6.9081) -> (3.9653, 6.9481) centre (0, 0) ccw
  line L97 (3.9653, 6.9481) -> (3.6162, 6.8546)
  arc A97 (3.6162, 6.8546) -> (3.5408, 6.8939) centre (0, 0) ccw
  line L98 (3.5408, 6.8939) -> (3.4172, 7.2335)
  arc A98 (3.4172, 7.2335) -> (3.3447, 7.2673) centre (0, 0) ccw
  line L99 (3.3447, 7.2673) -> (3.0051, 7.1437)
  arc A99 (3.0051, 7.1437) -> (2.9264, 7.1762) centre (0, 0) ccw
  line L100 (2.9264, 7.1762) -> (2.7737, 7.5038)
  arc A100 (2.7737, 7.5038) -> (2.6985, 7.5311) centre (0, 0) ccw
  line L101 (2.6985, 7.5311) -> (2.371, 7.3784)
  arc A101 (2.371, 7.3784) -> (2.2899, 7.404) centre (0, 0) ccw
  line L102 (2.2899, 7.404) -> (2.1092, 7.717)
  arc A102 (2.1092, 7.717) -> (2.0319, 7.7377) centre (0, 0) ccw
  line L103 (2.0319, 7.7377) -> (1.7189, 7.557)
  arc A103 (1.7189, 7.557) -> (1.6358, 7.5754) centre (0, 0) ccw
  line L104 (1.6358, 7.5754) -> (1.4286, 7.8714)
  arc A104 (1.4286, 7.8714) -> (1.3498, 7.8853) centre (0, 0) ccw
  line L105 (1.3498, 7.8853) -> (1.0537, 7.678)
  arc A105 (1.0537, 7.678) -> (0.9694, 7.6891) centre (0, 0) ccw
  line L106 (0.9694, 7.6891) -> (0.7371, 7.966)
  arc A106 (0.7371, 7.966) -> (0.6574, 7.9729) centre (0, 0) ccw
  line L107 (0.6574, 7.9729) -> (0.3806, 7.7407)
  arc A107 (0.3806, 7.7407) -> (0.2955, 7.7444) centre (0, 0) ccw
  line L108 (0.2955, 7.7444) -> (0.04, 7.9999)
  arc A108 (0.04, 7.9999) -> (-0.04, 7.9999) centre (0, 0) ccw
  line L109 (-0.04, 7.9999) -> (-0.2955, 7.7444)
  arc A109 (-0.2955, 7.7444) -> (-0.3806, 7.7407) centre (0, 0) ccw
  line L110 (-0.3806, 7.7407) -> (-0.6574, 7.9729)
  arc A110 (-0.6574, 7.9729) -> (-0.7371, 7.966) centre (0, 0) ccw
  line L111 (-0.7371, 7.966) -> (-0.9694, 7.6891)
  arc A111 (-0.9694, 7.6891) -> (-1.0537, 7.678) centre (0, 0) ccw
  line L112 (-1.0537, 7.678) -> (-1.3498, 7.8853)
  arc A112 (-1.3498, 7.8853) -> (-1.4286, 7.8714) centre (0, 0) ccw
  line L113 (-1.4286, 7.8714) -> (-1.6358, 7.5754)
  arc A113 (-1.6358, 7.5754) -> (-1.7189, 7.557) centre (0, 0) ccw
  line L114 (-1.7189, 7.557) -> (-2.0319, 7.7377)
  arc A114 (-2.0319, 7.7377) -> (-2.1092, 7.717) centre (0, 0) ccw
  line L115 (-2.1092, 7.717) -> (-2.2899, 7.404)
  arc A115 (-2.2899, 7.404) -> (-2.371, 7.3784) centre (0, 0) ccw
  line L116 (-2.371, 7.3784) -> (-2.6985, 7.5311)
  arc A116 (-2.6985, 7.5311) -> (-2.7737, 7.5038) centre (0, 0) ccw
  line L117 (-2.7737, 7.5038) -> (-2.9264, 7.1762)
  arc A117 (-2.9264, 7.1762) -> (-3.0051, 7.1437) centre (0, 0) ccw
  line L118 (-3.0051, 7.1437) -> (-3.3447, 7.2673)
  arc A118 (-3.3447, 7.2673) -> (-3.4172, 7.2335) centre (0, 0) ccw
  line L119 (-3.4172, 7.2335) -> (-3.5408, 6.8939)
  arc A119 (-3.5408, 6.8939) -> (-3.6162, 6.8546) centre (0, 0) ccw
  line L120 (-3.6162, 6.8546) -> (-3.9653, 6.9481)
  arc A120 (-3.9653, 6.9481) -> (-4.0346, 6.9081) centre (0, 0) ccw
  line L121 (-4.0346, 6.9081) -> (-4.1281, 6.559)
  arc A121 (-4.1281, 6.559) -> (-4.1999, 6.5133) centre (0, 0) ccw
  line L122 (-4.1999, 6.5133) -> (-4.5558, 6.5761)
  arc A122 (-4.5558, 6.5761) -> (-4.6213, 6.5302) centre (0, 0) ccw
  line L123 (-4.6213, 6.5302) -> (-4.6841, 6.1743)
  arc A123 (-4.6841, 6.1743) -> (-4.7516, 6.1225) centre (0, 0) ccw
  line L124 (-4.7516, 6.1225) -> (-5.1116, 6.154)
  arc A124 (-5.1116, 6.154) -> (-5.1729, 6.1026) centre (0, 0) ccw
  line L125 (-5.1729, 6.1026) -> (-5.2044, 5.7426)
  arc A125 (-5.2044, 5.7426) -> (-5.2671, 5.6851) centre (0, 0) ccw
  line L126 (-5.2671, 5.6851) -> (-5.6285, 5.6851)
  arc A126 (-5.6285, 5.6851) -> (-5.6851, 5.6285) centre (0, 0) ccw
  line L127 (-5.6851, 5.6285) -> (-5.6851, 5.2671)
  arc A127 (-5.6851, 5.2671) -> (-5.7426, 5.2044) centre (0, 0) ccw
  line L128 (-5.7426, 5.2044) -> (-6.1026, 5.1729)
  arc A128 (-6.1026, 5.1729) -> (-6.154, 5.1116) centre (0, 0) ccw
  line L129 (-6.154, 5.1116) -> (-6.1225, 4.7516)
  arc A129 (-6.1225, 4.7516) -> (-6.1743, 4.6841) centre (0, 0) ccw
  line L130 (-6.1743, 4.6841) -> (-6.5302, 4.6213)
  arc A130 (-6.5302, 4.6213) -> (-6.5761, 4.5558) centre (0, 0) ccw
  line L131 (-6.5761, 4.5558) -> (-6.5133, 4.1999)
  arc A131 (-6.5133, 4.1999) -> (-6.559, 4.1281) centre (0, 0) ccw
  line L132 (-6.559, 4.1281) -> (-6.9081, 4.0346)
  arc A132 (-6.9081, 4.0346) -> (-6.9481, 3.9653) centre (0, 0) ccw
  line L133 (-6.9481, 3.9653) -> (-6.8546, 3.6162)
  arc A133 (-6.8546, 3.6162) -> (-6.8939, 3.5408) centre (0, 0) ccw
  line L134 (-6.8939, 3.5408) -> (-7.2335, 3.4172)
  arc A134 (-7.2335, 3.4172) -> (-7.2673, 3.3447) centre (0, 0) ccw
  line L135 (-7.2673, 3.3447) -> (-7.1437, 3.0051)
  arc A135 (-7.1437, 3.0051) -> (-7.1762, 2.9264) centre (0, 0) ccw
  line L136 (-7.1762, 2.9264) -> (-7.5038, 2.7737)
  arc A136 (-7.5038, 2.7737) -> (-7.5311, 2.6985) centre (0, 0) ccw
  line L137 (-7.5311, 2.6985) -> (-7.3784, 2.371)
  arc A137 (-7.3784, 2.371) -> (-7.404, 2.2899) centre (0, 0) ccw
  line L138 (-7.404, 2.2899) -> (-7.717, 2.1092)
  arc A138 (-7.717, 2.1092) -> (-7.7377, 2.0319) centre (0, 0) ccw
  line L139 (-7.7377, 2.0319) -> (-7.557, 1.7189)
  arc A139 (-7.557, 1.7189) -> (-7.5754, 1.6358) centre (0, 0) ccw
  line L140 (-7.5754, 1.6358) -> (-7.8714, 1.4286)
  arc A140 (-7.8714, 1.4286) -> (-7.8853, 1.3498) centre (0, 0) ccw
  line L141 (-7.8853, 1.3498) -> (-7.678, 1.0537)
  arc A141 (-7.678, 1.0537) -> (-7.6891, 0.9694) centre (0, 0) ccw
  line L142 (-7.6891, 0.9694) -> (-7.966, 0.7371)
  arc A142 (-7.966, 0.7371) -> (-7.9729, 0.6574) centre (0, 0) ccw
  line L143 (-7.9729, 0.6574) -> (-7.7407, 0.3806)
  arc A143 (-7.7407, 0.3806) -> (-7.7444, 0.2955) centre (0, 0) ccw
  circle A144 centre (0, 0) radius 5.5
  dimension "d11" = 11
  constraint coincident A0.centre A1.centre
  measures "d11" diameter of A144
extrude "Extrude1" cut sketch "Sketch1 (1)" against normal blind 1 contours A144 bodies 1 in component "Knob"
sketch "Sketch2" plane through (0, 0, 0.9) normal (0, 0, 1) x (-1, 0, 0) in component "Knob"
  circle A0 centre (0, 0) radius 5.5
  line L0 (0.625, -4) -> (-0.625, -4)
  line L1 (-0.625, -4) -> (-0.625, -1.75)
  line L2 (-0.625, -1.75) -> (0.625, -1.75)
  line L3 (0.625, -1.75) -> (0.625, -4)
  line L4 (0, 0) -> (0, -1.75) construction
  dimension "d14" = 1.25
  dimension "d15" = 2.25
  dimension "d53" = 4
  constraint horizontal L0
  constraint vertical L1
  constraint horizontal L2
  constraint vertical L3
  constraint coincident A0.centre L4.start
  constraint midpoint L2 L4.end
  constraint perpendicular L2 L4
  measures "d14" distance of L1.end L2.end
  measures "d15" distance of L0 L2
  measures "d53" distance of L0 A0.centre
extrude "Extrude2'" cut sketch "Sketch2" against normal through all contours L0 L1 L2 L3 bodies 1 in component "Knob"
sketch "Sketch3" plane through (0, 0, 0) normal (0, 0, -1) x (1, 0, 0) in component "Knob"
  line L0 (-0.625, -4) -> (-0.625, -1.75)
  line L1 (-0.625, -1.75) -> (0.625, -1.75)
  line L2 (0.625, -1.75) -> (0.625, -4)
  line L3 (0.625, -4) -> (-0.625, -4)
  line L4 (7.9999, 0.04) -> (7.7444, 0.2955)
  arc A0 (7.7444, 0.2955) -> (7.7407, 0.3806) centre (0, 0) ccw
  line L5 (7.7407, 0.3806) -> (7.9729, 0.6574)
  arc A1 (7.9729, 0.6574) -> (7.966, 0.7371) centre (0, 0) ccw
  line L6 (7.966, 0.7371) -> (7.6891, 0.9694)
  arc A2 (7.6891, 0.9694) -> (7.678, 1.0537) centre (0, 0) ccw
  line L7 (7.678, 1.0537) -> (7.8853, 1.3498)
  arc A3 (7.8853, 1.3498) -> (7.8714, 1.4286) centre (0, 0) ccw
  line L8 (7.8714, 1.4286) -> (7.5754, 1.6358)
  arc A4 (7.5754, 1.6358) -> (7.557, 1.7189) centre (0, 0) ccw
  line L9 (7.557, 1.7189) -> (7.7377, 2.0319)
  arc A5 (7.7377, 2.0319) -> (7.717, 2.1092) centre (0, 0) ccw
  line L10 (7.717, 2.1092) -> (7.404, 2.2899)
  arc A6 (7.404, 2.2899) -> (7.3784, 2.371) centre (0, 0) ccw
  line L11 (7.3784, 2.371) -> (7.5311, 2.6985)
  arc A7 (7.5311, 2.6985) -> (7.5038, 2.7737) centre (0, 0) ccw
  line L12 (7.5038, 2.7737) -> (7.1762, 2.9264)
  arc A8 (7.1762, 2.9264) -> (7.1437, 3.0051) centre (0, 0) ccw
  line L13 (7.1437, 3.0051) -> (7.2673, 3.3447)
  arc A9 (7.2673, 3.3447) -> (7.2335, 3.4172) centre (0, 0) ccw
  line L14 (7.2335, 3.4172) -> (6.8939, 3.5408)
  arc A10 (6.8939, 3.5408) -> (6.8546, 3.6162) centre (0, 0) ccw
  line L15 (6.8546, 3.6162) -> (6.9481, 3.9653)
  arc A11 (6.9481, 3.9653) -> (6.9081, 4.0346) centre (0, 0) ccw
  line L16 (6.9081, 4.0346) -> (6.559, 4.1281)
  arc A12 (6.559, 4.1281) -> (6.5133, 4.1999) centre (0, 0) ccw
  line L17 (6.5133, 4.1999) -> (6.5761, 4.5558)
  arc A13 (6.5761, 4.5558) -> (6.5302, 4.6213) centre (0, 0) ccw
  line L18 (6.5302, 4.6213) -> (6.1743, 4.6841)
  arc A14 (6.1743, 4.6841) -> (6.1225, 4.7516) centre (0, 0) ccw
  line L19 (6.1225, 4.7516) -> (6.154, 5.1116)
  arc A15 (6.154, 5.1116) -> (6.1026, 5.1729) centre (0, 0) ccw
  line L20 (6.1026, 5.1729) -> (5.7426, 5.2044)
  arc A16 (5.7426, 5.2044) -> (5.6851, 5.2671) centre (0, 0) ccw
  line L21 (5.6851, 5.2671) -> (5.6851, 5.6285)
  arc A17 (5.6851, 5.6285) -> (5.6285, 5.6851) centre (0, 0) ccw
  line L22 (5.6285, 5.6851) -> (5.2671, 5.6851)
  arc A18 (5.2671, 5.6851) -> (5.2044, 5.7426) centre (0, 0) ccw
  line L23 (5.2044, 5.7426) -> (5.1729, 6.1026)
  arc A19 (5.1729, 6.1026) -> (5.1116, 6.154) centre (0, 0) ccw
  line L24 (5.1116, 6.154) -> (4.7516, 6.1225)
  arc A20 (4.7516, 6.1225) -> (4.6841, 6.1743) centre (0, 0) ccw
  line L25 (4.6841, 6.1743) -> (4.6213, 6.5302)
  arc A21 (4.6213, 6.5302) -> (4.5558, 6.5761) centre (0, 0) ccw
  line L26 (4.5558, 6.5761) -> (4.1999, 6.5133)
  arc A22 (4.1999, 6.5133) -> (4.1281, 6.559) centre (0, 0) ccw
  line L27 (4.1281, 6.559) -> (4.0346, 6.9081)
  arc A23 (4.0346, 6.9081) -> (3.9653, 6.9481) centre (0, 0) ccw
  line L28 (3.9653, 6.9481) -> (3.6162, 6.8546)
  arc A24 (3.6162, 6.8546) -> (3.5408, 6.8939) centre (0, 0) ccw
  line L29 (3.5408, 6.8939) -> (3.4172, 7.2335)
  arc A25 (3.4172, 7.2335) -> (3.3447, 7.2673) centre (0, 0) ccw
  line L30 (3.3447, 7.2673) -> (3.0051, 7.1437)
  arc A26 (3.0051, 7.1437) -> (2.9264, 7.1762) centre (0, 0) ccw
  line L31 (2.9264, 7.1762) -> (2.7737, 7.5038)
  arc A27 (2.7737, 7.5038) -> (2.6985, 7.5311) centre (0, 0) ccw
  line L32 (2.6985, 7.5311) -> (2.371, 7.3784)
  arc A28 (2.371, 7.3784) -> (2.2899, 7.404) centre (0, 0) ccw
  line L33 (2.2899, 7.404) -> (2.1092, 7.717)
  arc A29 (2.1092, 7.717) -> (2.0319, 7.7377) centre (0, 0) ccw
  line L34 (2.0319, 7.7377) -> (1.7189, 7.557)
  arc A30 (1.7189, 7.557) -> (1.6358, 7.5754) centre (0, 0) ccw
  line L35 (1.6358, 7.5754) -> (1.4286, 7.8714)
  arc A31 (1.4286, 7.8714) -> (1.3498, 7.8853) centre (0, 0) ccw
  line L36 (1.3498, 7.8853) -> (1.0537, 7.678)
  arc A32 (1.0537, 7.678) -> (0.9694, 7.6891) centre (0, 0) ccw
  line L37 (0.9694, 7.6891) -> (0.7371, 7.966)
  arc A33 (0.7371, 7.966) -> (0.6574, 7.9729) centre (0, 0) ccw
  line L38 (0.6574, 7.9729) -> (0.3806, 7.7407)
  arc A34 (0.3806, 7.7407) -> (0.2955, 7.7444) centre (0, 0) ccw
  line L39 (0.2955, 7.7444) -> (0.04, 7.9999)
  arc A35 (0.04, 7.9999) -> (-0.04, 7.9999) centre (0, 0) ccw
  line L40 (-0.04, 7.9999) -> (-0.2955, 7.7444)
  arc A36 (-0.2955, 7.7444) -> (-0.3806, 7.7407) centre (0, 0) ccw
  line L41 (-0.3806, 7.7407) -> (-0.6574, 7.9729)
  arc A37 (-0.6574, 7.9729) -> (-0.7371, 7.966) centre (0, 0) ccw
  line L42 (-0.7371, 7.966) -> (-0.9694, 7.6891)
  arc A38 (-0.9694, 7.6891) -> (-1.0537, 7.678) centre (0, 0) ccw
  line L43 (-1.0537, 7.678) -> (-1.3498, 7.8853)
  arc A39 (-1.3498, 7.8853) -> (-1.4286, 7.8714) centre (0, 0) ccw
  line L44 (-1.4286, 7.8714) -> (-1.6358, 7.5754)
  arc A40 (-1.6358, 7.5754) -> (-1.7189, 7.557) centre (0, 0) ccw
  line L45 (-1.7189, 7.557) -> (-2.0319, 7.7377)
  arc A41 (-2.0319, 7.7377) -> (-2.1092, 7.717) centre (0, 0) ccw
  line L46 (-2.1092, 7.717) -> (-2.2899, 7.404)
  arc A42 (-2.2899, 7.404) -> (-2.371, 7.3784) centre (0, 0) ccw
  line L47 (-2.371, 7.3784) -> (-2.6985, 7.5311)
  arc A43 (-2.6985, 7.5311) -> (-2.7737, 7.5038) centre (0, 0) ccw
  line L48 (-2.7737, 7.5038) -> (-2.9264, 7.1762)
  arc A44 (-2.9264, 7.1762) -> (-3.0051, 7.1437) centre (0, 0) ccw
  line L49 (-3.0051, 7.1437) -> (-3.3447, 7.2673)
  arc A45 (-3.3447, 7.2673) -> (-3.4172, 7.2335) centre (0, 0) ccw
  line L50 (-3.4172, 7.2335) -> (-3.5408, 6.8939)
  arc A46 (-3.5408, 6.8939) -> (-3.6162, 6.8546) centre (0, 0) ccw
  line L51 (-3.6162, 6.8546) -> (-3.9653, 6.9481)
  arc A47 (-3.9653, 6.9481) -> (-4.0346, 6.9081) centre (0, 0) ccw
  line L52 (-4.0346, 6.9081) -> (-4.1281, 6.559)
  arc A48 (-4.1281, 6.559) -> (-4.1999, 6.5133) centre (0, 0) ccw
  line L53 (-4.1999, 6.5133) -> (-4.5558, 6.5761)
  arc A49 (-4.5558, 6.5761) -> (-4.6213, 6.5302) centre (0, 0) ccw
  line L54 (-4.6213, 6.5302) -> (-4.6841, 6.1743)
  arc A50 (-4.6841, 6.1743) -> (-4.7516, 6.1225) centre (0, 0) ccw
  line L55 (-4.7516, 6.1225) -> (-5.1116, 6.154)
  arc A51 (-5.1116, 6.154) -> (-5.1729, 6.1026) centre (0, 0) ccw
  line L56 (-5.1729, 6.1026) -> (-5.2044, 5.7426)
  arc A52 (-5.2044, 5.7426) -> (-5.2671, 5.6851) centre (0, 0) ccw
  line L57 (-5.2671, 5.6851) -> (-5.6285, 5.6851)
  arc A53 (-5.6285, 5.6851) -> (-5.6851, 5.6285) centre (0, 0) ccw
  line L58 (-5.6851, 5.6285) -> (-5.6851, 5.2671)
  arc A54 (-5.6851, 5.2671) -> (-5.7426, 5.2044) centre (0, 0) ccw
  line L59 (-5.7426, 5.2044) -> (-6.1026, 5.1729)
  arc A55 (-6.1026, 5.1729) -> (-6.154, 5.1116) centre (0, 0) ccw
  line L60 (-6.154, 5.1116) -> (-6.1225, 4.7516)
  arc A56 (-6.1225, 4.7516) -> (-6.1743, 4.6841) centre (0, 0) ccw
  line L61 (-6.1743, 4.6841) -> (-6.5302, 4.6213)
  arc A57 (-6.5302, 4.6213) -> (-6.5761, 4.5558) centre (0, 0) ccw
  line L62 (-6.5761, 4.5558) -> (-6.5133, 4.1999)
  arc A58 (-6.5133, 4.1999) -> (-6.559, 4.1281) centre (0, 0) ccw
  line L63 (-6.559, 4.1281) -> (-6.9081, 4.0346)
  arc A59 (-6.9081, 4.0346) -> (-6.9481, 3.9653) centre (0, 0) ccw
  line L64 (-6.9481, 3.9653) -> (-6.8546, 3.6162)
  arc A60 (-6.8546, 3.6162) -> (-6.8939, 3.5408) centre (0, 0) ccw
  line L65 (-6.8939, 3.5408) -> (-7.2335, 3.4172)
  arc A61 (-7.2335, 3.4172) -> (-7.2673, 3.3447) centre (0, 0) ccw
  line L66 (-7.2673, 3.3447) -> (-7.1437, 3.0051)
  arc A62 (-7.1437, 3.0051) -> (-7.1762, 2.9264) centre (0, 0) ccw
  line L67 (-7.1762, 2.9264) -> (-7.5038, 2.7737)
  arc A63 (-7.5038, 2.7737) -> (-7.5311, 2.6985) centre (0, 0) ccw
  line L68 (-7.5311, 2.6985) -> (-7.3784, 2.371)
  arc A64 (-7.3784, 2.371) -> (-7.404, 2.2899) centre (0, 0) ccw
  line L69 (-7.404, 2.2899) -> (-7.717, 2.1092)
  arc A65 (-7.717, 2.1092) -> (-7.7377, 2.0319) centre (0, 0) ccw
  line L70 (-7.7377, 2.0319) -> (-7.557, 1.7189)
  arc A66 (-7.557, 1.7189) -> (-7.5754, 1.6358) centre (0, 0) ccw
  line L71 (-7.5754, 1.6358) -> (-7.8714, 1.4286)
  arc A67 (-7.8714, 1.4286) -> (-7.8853, 1.3498) centre (0, 0) ccw
  line L72 (-7.8853, 1.3498) -> (-7.678, 1.0537)
  arc A68 (-7.678, 1.0537) -> (-7.6891, 0.9694) centre (0, 0) ccw
  line L73 (-7.6891, 0.9694) -> (-7.966, 0.7371)
  arc A69 (-7.966, 0.7371) -> (-7.9729, 0.6574) centre (0, 0) ccw
  line L74 (-7.9729, 0.6574) -> (-7.7407, 0.3806)
  arc A70 (-7.7407, 0.3806) -> (-7.7444, 0.2955) centre (0, 0) ccw
  line L75 (-7.7444, 0.2955) -> (-7.9999, 0.04)
  arc A71 (-7.9999, 0.04) -> (-7.9999, -0.04) centre (0, 0) ccw
  line L76 (-7.9999, -0.04) -> (-7.7444, -0.2955)
  arc A72 (-7.7444, -0.2955) -> (-7.7407, -0.3806) centre (0, 0) ccw
  line L77 (-7.7407, -0.3806) -> (-7.9729, -0.6574)
  arc A73 (-7.9729, -0.6574) -> (-7.966, -0.7371) centre (0, 0) ccw
  line L78 (-7.966, -0.7371) -> (-7.6891, -0.9694)
  arc A74 (-7.6891, -0.9694) -> (-7.678, -1.0537) centre (0, 0) ccw
  line L79 (-7.678, -1.0537) -> (-7.8853, -1.3498)
  arc A75 (-7.8853, -1.3498) -> (-7.8714, -1.4286) centre (0, 0) ccw
  line L80 (-7.8714, -1.4286) -> (-7.5754, -1.6358)
  arc A76 (-7.5754, -1.6358) -> (-7.557, -1.7189) centre (0, 0) ccw
  line L81 (-7.557, -1.7189) -> (-7.7377, -2.0319)
  arc A77 (-7.7377, -2.0319) -> (-7.717, -2.1092) centre (0, 0) ccw
  line L82 (-7.717, -2.1092) -> (-7.404, -2.2899)
  arc A78 (-7.404, -2.2899) -> (-7.3784, -2.371) centre (0, 0) ccw
  line L83 (-7.3784, -2.371) -> (-7.5311, -2.6985)
  arc A79 (-7.5311, -2.6985) -> (-7.5038, -2.7737) centre (0, 0) ccw
  line L84 (-7.5038, -2.7737) -> (-7.1762, -2.9264)
  arc A80 (-7.1762, -2.9264) -> (-7.1437, -3.0051) centre (0, 0) ccw
  line L85 (-7.1437, -3.0051) -> (-7.2673, -3.3447)
  arc A81 (-7.2673, -3.3447) -> (-7.2335, -3.4172) centre (0, 0) ccw
  line L86 (-7.2335, -3.4172) -> (-6.8939, -3.5408)
  arc A82 (-6.8939, -3.5408) -> (-6.8546, -3.6162) centre (0, 0) ccw
  line L87 (-6.8546, -3.6162) -> (-6.9481, -3.9653)
  arc A83 (-6.9481, -3.9653) -> (-6.9081, -4.0346) centre (0, 0) ccw
  line L88 (-6.9081, -4.0346) -> (-6.559, -4.1281)
  arc A84 (-6.559, -4.1281) -> (-6.5133, -4.1999) centre (0, 0) ccw
  line L89 (-6.5133, -4.1999) -> (-6.5761, -4.5558)
  arc A85 (-6.5761, -4.5558) -> (-6.5302, -4.6213) centre (0, 0) ccw
  line L90 (-6.5302, -4.6213) -> (-6.1743, -4.6841)
  arc A86 (-6.1743, -4.6841) -> (-6.1225, -4.7516) centre (0, 0) ccw
  line L91 (-6.1225, -4.7516) -> (-6.154, -5.1116)
  arc A87 (-6.154, -5.1116) -> (-6.1026, -5.1729) centre (0, 0) ccw
  line L92 (-6.1026, -5.1729) -> (-5.7426, -5.2044)
  arc A88 (-5.7426, -5.2044) -> (-5.6851, -5.2671) centre (0, 0) ccw
  line L93 (-5.6851, -5.2671) -> (-5.6851, -5.6285)
  arc A89 (-5.6851, -5.6285) -> (-5.6285, -5.6851) centre (0, 0) ccw
  line L94 (-5.6285, -5.6851) -> (-5.2671, -5.6851)
  arc A90 (-5.2671, -5.6851) -> (-5.2044, -5.7426) centre (0, 0) ccw
  line L95 (-5.2044, -5.7426) -> (-5.1729, -6.1026)
  arc A91 (-5.1729, -6.1026) -> (-5.1116, -6.154) centre (0, 0) ccw
  line L96 (-5.1116, -6.154) -> (-4.7516, -6.1225)
  arc A92 (-4.7516, -6.1225) -> (-4.6841, -6.1743) centre (0, 0) ccw
  line L97 (-4.6841, -6.1743) -> (-4.6213, -6.5302)
  arc A93 (-4.6213, -6.5302) -> (-4.5558, -6.5761) centre (0, 0) ccw
  line L98 (-4.5558, -6.5761) -> (-4.1999, -6.5133)
  arc A94 (-4.1999, -6.5133) -> (-4.1281, -6.559) centre (0, 0) ccw
  line L99 (-4.1281, -6.559) -> (-4.0346, -6.9081)
  arc A95 (-4.0346, -6.9081) -> (-3.9653, -6.9481) centre (0, 0) ccw
  line L100 (-3.9653, -6.9481) -> (-3.6162, -6.8546)
  arc A96 (-3.6162, -6.8546) -> (-3.5408, -6.8939) centre (0, 0) ccw
  line L101 (-3.5408, -6.8939) -> (-3.4172, -7.2335)
  arc A97 (-3.4172, -7.2335) -> (-3.3447, -7.2673) centre (0, 0) ccw
  line L102 (-3.3447, -7.2673) -> (-3.0051, -7.1437)
  arc A98 (-3.0051, -7.1437) -> (-2.9264, -7.1762) centre (0, 0) ccw
  line L103 (-2.9264, -7.1762) -> (-2.7737, -7.5038)
  arc A99 (-2.7737, -7.5038) -> (-2.6985, -7.5311) centre (0, 0) ccw
  line L104 (-2.6985, -7.5311) -> (-2.371, -7.3784)
  arc A100 (-2.371, -7.3784) -> (-2.2899, -7.404) centre (0, 0) ccw
  line L105 (-2.2899, -7.404) -> (-2.1092, -7.717)
  arc A101 (-2.1092, -7.717) -> (-2.0319, -7.7377) centre (0, 0) ccw
  line L106 (-2.0319, -7.7377) -> (-1.7189, -7.557)
  arc A102 (-1.7189, -7.557) -> (-1.6358, -7.5754) centre (0, 0) ccw
  line L107 (-1.6358, -7.5754) -> (-1.4286, -7.8714)
  arc A103 (-1.4286, -7.8714) -> (-1.3498, -7.8853) centre (0, 0) ccw
  line L108 (-1.3498, -7.8853) -> (-1.0537, -7.678)
  arc A104 (-1.0537, -7.678) -> (-0.9694, -7.6891) centre (0, 0) ccw
  line L109 (-0.9694, -7.6891) -> (-0.7371, -7.966)
  arc A105 (-0.7371, -7.966) -> (-0.6574, -7.9729) centre (0, 0) ccw
  line L110 (-0.6574, -7.9729) -> (-0.3806, -7.7407)
  arc A106 (-0.3806, -7.7407) -> (-0.2955, -7.7444) centre (0, 0) ccw
  line L111 (-0.2955, -7.7444) -> (-0.04, -7.9999)
  arc A107 (-0.04, -7.9999) -> (0.04, -7.9999) centre (0, 0) ccw
  line L112 (0.04, -7.9999) -> (0.2955, -7.7444)
  arc A108 (0.2955, -7.7444) -> (0.3806, -7.7407) centre (0, 0) ccw
  line L113 (0.3806, -7.7407) -> (0.6574, -7.9729)
  arc A109 (0.6574, -7.9729) -> (0.7371, -7.966) centre (0, 0) ccw
  line L114 (0.7371, -7.966) -> (0.9694, -7.6891)
  arc A110 (0.9694, -7.6891) -> (1.0537, -7.678) centre (0, 0) ccw
  line L115 (1.0537, -7.678) -> (1.3498, -7.8853)
  arc A111 (1.3498, -7.8853) -> (1.4286, -7.8714) centre (0, 0) ccw
  line L116 (1.4286, -7.8714) -> (1.6358, -7.5754)
  arc A112 (1.6358, -7.5754) -> (1.7189, -7.557) centre (0, 0) ccw
  line L117 (1.7189, -7.557) -> (2.0319, -7.7377)
  arc A113 (2.0319, -7.7377) -> (2.1092, -7.717) centre (0, 0) ccw
  line L118 (2.1092, -7.717) -> (2.2899, -7.404)
  arc A114 (2.2899, -7.404) -> (2.371, -7.3784) centre (0, 0) ccw
  line L119 (2.371, -7.3784) -> (2.6985, -7.5311)
  arc A115 (2.6985, -7.5311) -> (2.7737, -7.5038) centre (0, 0) ccw
  line L120 (2.7737, -7.5038) -> (2.9264, -7.1762)
  arc A116 (2.9264, -7.1762) -> (3.0051, -7.1437) centre (0, 0) ccw
  line L121 (3.0051, -7.1437) -> (3.3447, -7.2673)
  arc A117 (3.3447, -7.2673) -> (3.4172, -7.2335) centre (0, 0) ccw
  line L122 (3.4172, -7.2335) -> (3.5408, -6.8939)
  arc A118 (3.5408, -6.8939) -> (3.6162, -6.8546) centre (0, 0) ccw
  line L123 (3.6162, -6.8546) -> (3.9653, -6.9481)
  arc A119 (3.9653, -6.9481) -> (4.0346, -6.9081) centre (0, 0) ccw
  line L124 (4.0346, -6.9081) -> (4.1281, -6.559)
  arc A120 (4.1281, -6.559) -> (4.1999, -6.5133) centre (0, 0) ccw
  line L125 (4.1999, -6.5133) -> (4.5558, -6.5761)
  arc A121 (4.5558, -6.5761) -> (4.6213, -6.5302) centre (0, 0) ccw
  line L126 (4.6213, -6.5302) -> (4.6841, -6.1743)
  arc A122 (4.6841, -6.1743) -> (4.7516, -6.1225) centre (0, 0) ccw
  line L127 (4.7516, -6.1225) -> (5.1116, -6.154)
  arc A123 (5.1116, -6.154) -> (5.1729, -6.1026) centre (0, 0) ccw
  line L128 (5.1729, -6.1026) -> (5.2044, -5.7426)
  arc A124 (5.2044, -5.7426) -> (5.2671, -5.6851) centre (0, 0) ccw
  line L129 (5.2671, -5.6851) -> (5.6285, -5.6851)
  arc A125 (5.6285, -5.6851) -> (5.6851, -5.6285) centre (0, 0) ccw
  line L130 (5.6851, -5.6285) -> (5.6851, -5.2671)
  arc A126 (5.6851, -5.2671) -> (5.7426, -5.2044) centre (0, 0) ccw
  line L131 (5.7426, -5.2044) -> (6.1026, -5.1729)
  arc A127 (6.1026, -5.1729) -> (6.154, -5.1116) centre (0, 0) ccw
  line L132 (6.154, -5.1116) -> (6.1225, -4.7516)
  arc A128 (6.1225, -4.7516) -> (6.1743, -4.6841) centre (0, 0) ccw
  line L133 (6.1743, -4.6841) -> (6.5302, -4.6213)
  arc A129 (6.5302, -4.6213) -> (6.5761, -4.5558) centre (0, 0) ccw
  line L134 (6.5761, -4.5558) -> (6.5133, -4.1999)
  arc A130 (6.5133, -4.1999) -> (6.559, -4.1281) centre (0, 0) ccw
  line L135 (6.559, -4.1281) -> (6.9081, -4.0346)
  arc A131 (6.9081, -4.0346) -> (6.9481, -3.9653) centre (0, 0) ccw
  line L136 (6.9481, -3.9653) -> (6.8546, -3.6162)
  arc A132 (6.8546, -3.6162) -> (6.8939, -3.5408) centre (0, 0) ccw
  line L137 (6.8939, -3.5408) -> (7.2335, -3.4172)
  arc A133 (7.2335, -3.4172) -> (7.2673, -3.3447) centre (0, 0) ccw
  line L138 (7.2673, -3.3447) -> (7.1437, -3.0051)
  arc A134 (7.1437, -3.0051) -> (7.1762, -2.9264) centre (0, 0) ccw
  line L139 (7.1762, -2.9264) -> (7.5038, -2.7737)
  arc A135 (7.5038, -2.7737) -> (7.5311, -2.6985) centre (0, 0) ccw
  line L140 (7.5311, -2.6985) -> (7.3784, -2.371)
  arc A136 (7.3784, -2.371) -> (7.404, -2.2899) centre (0, 0) ccw
  line L141 (7.404, -2.2899) -> (7.717, -2.1092)
  arc A137 (7.717, -2.1092) -> (7.7377, -2.0319) centre (0, 0) ccw
  line L142 (7.7377, -2.0319) -> (7.557, -1.7189)
  arc A138 (7.557, -1.7189) -> (7.5754, -1.6358) centre (0, 0) ccw
  line L143 (7.5754, -1.6358) -> (7.8714, -1.4286)
  arc A139 (7.8714, -1.4286) -> (7.8853, -1.3498) centre (0, 0) ccw
  line L144 (7.8853, -1.3498) -> (7.678, -1.0537)
  arc A140 (7.678, -1.0537) -> (7.6891, -0.9694) centre (0, 0) ccw
  line L145 (7.6891, -0.9694) -> (7.966, -0.7371)
  arc A141 (7.966, -0.7371) -> (7.9729, -0.6574) centre (0, 0) ccw
  line L146 (7.9729, -0.6574) -> (7.7407, -0.3806)
  arc A142 (7.7407, -0.3806) -> (7.7444, -0.2955) centre (0, 0) ccw
  line L147 (7.7444, -0.2955) -> (7.9999, -0.04)
  arc A143 (7.9999, -0.04) -> (7.9999, 0.04) centre (0, 0) ccw
  circle A144 centre (0, 0) radius 5
  dimension "d18" = 10
  constraint concentric A0 A144
  measures "d18" diameter of A144
extrude "Extrude3" add sketch "Sketch3" along normal blind 0.7 contours L0 L1 L2 L3 | A144 bodies 1 in component "Knob"